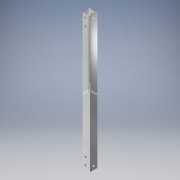
# Autodesk Inventor part: 15102898-16-P-0206
Saved by Autodesk Inventor 2017 (Build 210142000, 142)
## iProperties
Created: 2016-10-02
Part Number: 15102898-16-P-0206
Material: Aluminum 6061
Document SubType Name: Modeling
Designer: gus
Density: 2.7 g/cm^3
Appearance: Aluminum - Flat
Author: gus
Autodesk Inventor part; units mm, degrees
ref_plane "YZ Plane" through (0, 0, 0) normal (1, 0, 0) x (0, 1, 0)
ref_plane "XZ Plane" through (0, 0, 0) normal (0, 1, 0) x (-1, 0, 0)
ref_plane "XY Plane" through (0, 0, 0) normal (0, 0, 1) x (1, 0, 0)
sketch "Sketch1" plane through (0, 0, 0) normal (0, 1, 0) x (-1, 0, 0)
  line L0 (0, 0) -> (25.4, 0)
  line L1 (25.4, 0) -> (25.4, 25.4)
  line L2 (25.4, 25.4) -> (0, 25.4)
  line L3 (0, 25.4) -> (0, 0)
  line L4 (22.225, 22.225) -> (22.225, 3.175)
  line L5 (22.225, 3.175) -> (3.175, 3.175)
  line L6 (3.175, 3.175) -> (3.175, 22.225)
  line L7 (3.175, 22.225) -> (22.225, 22.225)
  dimension "d0" = 25.4
  dimension "d1" = 25.4
  dimension "d2" = 3.175
  constraints: 16 end point, 4 parallel, 2 perpendicular, 1 horizontal, 3 other
  measures "d0" distance of L2.end L1.end
  measures "d1" distance of L1.end L0.end
  measures "d2" distance between parallel lines of L1 L4
extrude "Extrusion1" add sketch "Sketch1" along normal blind 472.9226
sketch "Sketch2" plane through (-25.4, 0, 0) normal (-1, 0, 0) x (0, 0, 1)
  circle A0 centre (12.7, 12.7) radius 3.175
  circle A1 centre (12.7, 460.2226) radius 3.175
  line L0 (22.225, 472.9226) -> (3.175, 472.9226) projected
  line L1 (25.4, 0) -> (25.4, 472.9226) projected
  line L2 (25.4, 0) -> (25.4, 472.9226) projected
  line L3 (0, 0) -> (25.4, 0) projected
  dimension "d5" = 6.35
  dimension "d6" = 6.35
  dimension "d7" = 12.7
  dimension "d8" = 12.7
  dimension "d9" = 12.7
  dimension "d10" = 12.7
  constraints: 2 centre point
  measures "d5" diameter of A0
  measures "d6" diameter of A1
  measures "d7" distance from line of L0 A1.centre
  measures "d8" distance from line of L1 A1.centre
  measures "d9" distance from line of A0.centre L2
  measures "d10" distance from line of L3 A0.centre
extrude "Extrusion2" cut sketch "Sketch2" against normal blind 25.4
sketch "Sketch3" plane through (-25.4, 0, 25.4) normal (0, 0, 1) x (1, 0, 0)
  circle A0 centre (9.525, 460.2226) radius 3.175
  circle A1 centre (9.525, 434.8226) radius 3.175
  line L0 (0, 472.9226) -> (25.4, 472.9226) projected
  line L1 (0, 0) -> (0, 472.9226) projected
  circle A2 centre (9.525, 12.7) radius 3.175
  circle A3 centre (9.525, 38.1) radius 3.175
  line L2 (0, 0) -> (25.4, 0) projected
  dimension "d13" = 12.7
  dimension "d14" = 9.525
  dimension "d15" = 9.525
  dimension "d16" = 6.35
  dimension "d17" = 38.1
  dimension "d18" = 6.35
  dimension "d19" = 6.35
  dimension "d20" = 9.525
  dimension "d21" = 9.525
  dimension "d22" = 38.1
  dimension "d23" = 12.7
  constraints: 4 centre point, 1 equal radius
  measures "d13" distance from line of A0.centre L0
  measures "d14" distance from line of L1 A1.centre
  measures "d15" distance from line of A0.centre L1
  measures "d16" diameter of A0
  measures "d17" distance from line of L0 A1.centre
  measures "d18" diameter of A2
  measures "d19" diameter of A3
  measures "d20" distance from line of L1 A3.centre
  measures "d21" distance from line of L1 A2.centre
  measures "d22" distance from line of L2 A3.centre
  measures "d23" distance from line of A2.centre L2
extrude "Extrusion3" cut sketch "Sketch3" against normal blind 25.4
body "Solid1"
